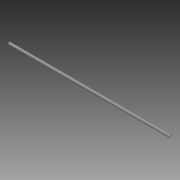
# Autodesk Inventor part: Plastic Tube (15.5)
Saved by Autodesk Inventor 2015 SP1 (Build 190203100, 203)
## iProperties
Created: 2014-10-09
Part Number: Plastic Tube (15.5)
Material: Generic
Document SubType Name: Modeling
Designer: Jordan M
Density: 1 g/cm^3
Appearance: Default
Author: Jordan M
Autodesk Inventor part; units mm, degrees
ref_plane "YZ Plane" through (0, 0, 0) normal (1, 0, 0) x (0, 1, 0)
ref_plane "XZ Plane" through (0, 0, 0) normal (0, 1, 0) x (-1, 0, 0)
ref_plane "XY Plane" through (0, 0, 0) normal (0, 0, 1) x (1, 0, 0)
sketch "Sketch1" plane through (0, 0, 0) normal (1, 0, 0) x (0, 1, 0)
  circle A0 centre (0, 0) radius 3.175
  dimension "d0" = 6.35
  constraints: 1 centre point, 1 coincident
  measures "d0" diameter of A0
extrude "Extrusion1" add sketch "Sketch1" along normal blind 393.7
hole "Hole1" at (393.7, -0.0197, 0.0328) direction (-1, 0, 0) diameter 5.08 end through all
body "Solid1"
